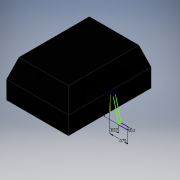
# Autodesk Inventor part: VO14642AT
Saved by Autodesk Inventor 2016 (Build 200138000, 138)
## iProperties
Created: 2016-08-10
Part Number: VO14642AT
Material: Generic
Document SubType Name: Modeling
Designer: jfixelle
Density: 1 g/cm^3
Appearance: Black
Author: jfixelle
Autodesk Inventor part; units mm, degrees
ref_plane "YZ Plane" through (0, 0, 0) normal (1, 0, 0) x (0, 1, 0)
ref_plane "XZ Plane" through (0, 0, 0) normal (0, 1, 0) x (-1, 0, 0)
ref_plane "XY Plane" through (0, 0, 0) normal (0, 0, 1) x (1, 0, 0)
sketch "Sketch1" plane through (0, 0, 0) normal (0, 1, 0) x (-1, 0, 0)
  line L0 (3.25, 4.35) -> (-3.25, 4.35)
  line L1 (-3.25, 4.35) -> (-3.25, -4.35)
  line L2 (-3.25, -4.35) -> (3.25, -4.35)
  line L3 (3.25, -4.35) -> (3.25, 4.35)
  point P0 (0, 0)
  dimension "d0" = 6.5
  dimension "d1" = 3.25
  dimension "d2" = 4.35
  dimension "d3" = 8.7
  constraints: 8 end point, 2 parallel, 1 horizontal, 1 perpendicular
  measures "d0" distance of L1.end L2.end
  measures "d1" distance from line of point (0, 0) L3
  measures "d2" distance from line of point (0, 0) L0
  measures "d3" distance of L2.end L0.start
extrude "Extrusion1" add sketch "Sketch1" along normal blind 3.9
chamfer "Chamfer1" distance 2 angle 18 1 edges at (3.25, 3.9, 0) measured on face at (3.25, 3.4, 0)
chamfer "Chamfer2" distance 2 angle 18 1 edges at (-0.3249, 3.9, 4.35) measured on face at (-0.3249, 3.4, 4.35)
chamfer "Chamfer3" distance 2 angle 18 1 edges at (-0.3249, 3.9, -4.35) measured on face at (-0.3249, 3.4, -4.35)
chamfer "Chamfer4" distance 2 angle 18 1 edges at (-3.25, 3.9, 0) measured on face at (-3.25, 3.4, 0)
sketch "Sketch2" plane through (0, 0, 0) normal (0, 0, 1) x (1, 0, 0)
  line L0 (3.25, 1.6) -> (3.25, 1.9)
  line L1 (3.25, 1.9) -> (3.81, 1.9)
  line L2 (3.81, 1.9) -> (4.4216, -0.4)
  line L3 (4.4216, -0.4) -> (5.15, -0.4)
  line L4 (5.15, -0.4) -> (5.15, -0.7)
  line L5 (5.15, -0.7) -> (4.2, -0.7)
  line L6 (4.2, -0.7) -> (3.5884, 1.6)
  line L7 (3.5884, 1.6) -> (3.25, 1.6)
  line L8 (3.25, 0) -> (3.25, 1.9) projected
  line L9 (-3.25, 0) -> (3.25, 0) projected
  line L10 (-3.25, 1.9) -> (3.25, 1.9) projected
  point P0 (0, 0)
  dimension "d18" = 0.3
  dimension "d19" = 0.3
  dimension "d20" = 0
  dimension "d21" = 0.95
  dimension "d22" = 1.9
  dimension "d23" = 0.7
  dimension "d24" = 0.56
  dimension "d25" = 0
  constraints: 16 end point, 3 parallel, 3 perpendicular, 1 vertical
  measures "d18" distance of L3.end L4.end
  measures "d19" distance of L0.start L0.end
  measures "d20" distance between parallel lines of L8 L0
  measures "d21" distance from line of L8 L5.end
  measures "d22" distance between parallel lines of L8 L4
  measures "d23" distance between parallel lines of L9 L5
  measures "d24" distance from line of L8 L1.end
  measures "d25" distance between parallel lines of L10 L1
body "Solid1"
